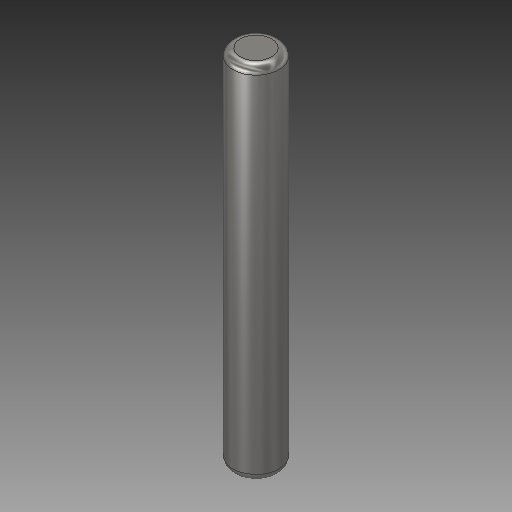
# Autodesk Inventor part: TestRod
Saved by Autodesk Inventor 2018 (Build 220112000, 112)
## iProperties
Created: 2017-10-21
Part Number: TestRod
Material: Steel, Carbon
Document SubType Name: Modeling
Designer: Bryce Richards
Density: 7.85 g/cm^3
Appearance: Semi-Polished
Mass: 747.474 g
Surface Area: 160.131 cm^2
Volume: 95.2196 cm^3
Author: Bryce Richards
Autodesk Inventor part; units mm, degrees
ref_plane "YZ Plane" through (0, 0, 0) normal (1, 0, 0) x (0, 1, 0)
ref_plane "XZ Plane" through (0, 0, 0) normal (0, 1, 0) x (-1, 0, 0)
ref_plane "XY Plane" through (0, 0, 0) normal (0, 0, 1) x (1, 0, 0)
sketch "Sketch1" plane through (0, 0, 0) normal (0, 1, 0) x (-1, 0, 0)
  circle A0 centre (0, 0) radius 12.5
  dimension "d0" = 25
  constraints: 1 centre point, 1 coincident
  measures "d0" diameter of A0
extrude "Extrusion1" add sketch "Sketch1" along normal blind 195
fillet "Fillet1" radius 4 2 edges at (12.5, 0, 0) (12.5, 195, 0)
body "Solid1"
